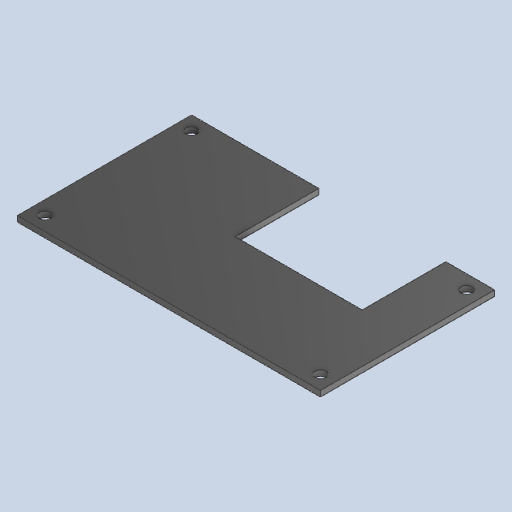
# Autodesk Inventor part: ExpansionBoard
Saved by Autodesk Inventor 2022.3 (Build 263350000, 350)
## iProperties
Part Number: ExpansionBoard
Material: 一般
Document SubType Name: Modeling
Designer: Masato Kubotera
Density: 1 g/cm^3
Appearance: 滑らか - 黒
Description: CircuitBoard
Mass: 5.60293 g
Surface Area: 75.832 cm^2
Volume: 5.60293 cm^3
Author: MasatoKubotera
Autodesk Inventor part; units mm, degrees
ref_plane "YZ Plane" through (0, 0, 0) normal (1, 0, 0) x (0, 1, 0)
ref_plane "XZ Plane" through (0, 0, 0) normal (0, 1, 0) x (-1, 0, 0)
ref_plane "XY Plane" through (0, 0, 0) normal (0, 0, 1) x (1, 0, 0)
derived "JetsonXavierNX_and_EN715.ipt"
sketch "スケッチ1" plane through (0, 0, 0) normal (0, 0, 1) x (1, 0, 0)
  line L0 (35.3, 43.5) -> (-35.3, 43.5)
  line L1 (-35.3, 43.5) -> (-35.3, -43.5)
  line L2 (-35.3, -43.5) -> (35.3, -43.5)
  line L3 (35.3, 43.5) -> (-35.3, -43.5) construction
  line L4 (-35.3, 43.5) -> (35.3, -43.5) construction
  circle A0 centre (-31.3, -39.5) radius 1.6
  circle A1 centre (10.7, -39.5) radius 1.6
  line L5 (29.7, 0) -> (-35.3, 0) construction
  circle A2 centre (10.7, 39.5) radius 1.6
  circle A3 centre (-31.3, 39.5) radius 1.6
  line L6 (14.65, 36.45) -> (-35.1, 36.45)
  line L7 (-35.1, 36.45) -> (-35.1, -36.45)
  line L8 (-35.1, -36.45) -> (14.65, -36.45)
  line L9 (14.65, -36.45) -> (14.65, 36.45)
  line L10 (14.65, 36.45) -> (-35.1, -36.45) construction
  line L11 (-35.1, 36.45) -> (14.65, -36.45) construction
  line L12 (35.3, -24) -> (29.7, -24)
  line L13 (29.7, -24) -> (29.7, 24)
  line L14 (29.7, 24) -> (35.3, 24)
  line L15 (35.3, -43.5) -> (35.3, -24)
  line L16 (35.3, 24) -> (35.3, 43.5)
  line L17 (4.4, 28.9) -> (-34.6, 28.9)
  line L18 (-34.6, 28.9) -> (-34.6, -28.9)
  line L19 (-34.6, -28.9) -> (4.4, -28.9)
  line L20 (4.4, -28.9) -> (4.4, 28.9)
  line L21 (4.4, 28.9) -> (-34.6, -28.9) construction
  line L22 (-34.6, 28.9) -> (4.4, -28.9) construction
  line L23 (-35.3, 11.2) -> (-12.8, 11.2)
  line L24 (-12.8, 11.2) -> (-12.8, 28)
  line L25 (-12.8, 28) -> (-35.3, 28)
  line L26 (-35.3, 11.2) -> (-37.8, 11.2)
  line L27 (-37.8, 11.2) -> (-37.8, 28)
  line L28 (-37.8, 28) -> (-35.3, 28)
  line L29 (-36.3, 7.17) -> (-19.3, 7.17)
  line L30 (-19.3, 7.17) -> (-19.3, -5.93)
  line L31 (-19.3, -5.93) -> (-36.3, -5.93)
  line L32 (-36.3, -5.93) -> (-36.3, 7.17)
  line L33 (-36.3, -12.41) -> (-25.3, -12.41)
  line L34 (-25.3, -12.41) -> (-25.3, -28.01)
  line L35 (-25.3, -28.01) -> (-36.3, -28.01)
  line L36 (-36.3, -28.01) -> (-36.3, -12.41)
  point P0 (0, 0)
  point P1 (-10.225, 0)
  point P2 (-10.225, 0)
  point P3 (-15.1, 0)
sketch "スケッチ2" plane through (0, 0, 0) normal (0, 0, 1) x (1, 0, 0)
  line L0 (-35.3, 43.5) -> (14.7, 43.5)
  line L1 (14.7, 43.5) -> (14.7, -43.5)
  line L2 (14.7, -43.5) -> (-35.3, -43.5)
  circle A0 centre (-31.3, 39.5) radius 1.6 projected
  circle A1 centre (10.7, 39.5) radius 1.6 projected
  circle A2 centre (-31.3, -39.5) radius 1.6 projected
  circle A3 centre (10.7, -39.5) radius 1.6 projected
  line L3 (-35.3, 29.5) -> (-11.3, 29.5)
  line L4 (-11.3, 29.5) -> (-11.3, -7)
  line L5 (-11.3, -7) -> (-35.3, -7)
  line L6 (-35.3, -43.5) -> (-35.3, -7)
  line L7 (-35.3, 29.5) -> (-35.3, 43.5)
  point P0 (0, 0)
  dimension "d1" = 4
  dimension "d2" = 4
  dimension "d3" = 14
  dimension "d4" = 36.5
  dimension "d5" = 36.5
  dimension "d6" = 24
  constraints: 16 end point, 5 parallel, 3 perpendicular, 2 coincident, 2 horizontal
  measures "d1" horizontal distance of L0.start A0.centre
  measures "d2" horizontal distance of A1.centre L0.end
  measures "d3" distance of L3.start L0.start
  measures "d4" distance of L2.end L5.end
  measures "d5" distance of L3.end L4.end
  measures "d6" distance of L3.start L3.end
extrude "押し出し1" add sketch "スケッチ2" along normal blind 1.6
equation "\"d2\" = d1"
